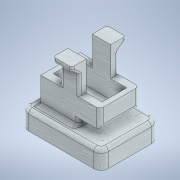
# Autodesk Inventor part: ramie 03-2
Saved by Autodesk Inventor 2021 (Build 250183000, 183)
## iProperties
Created: 2021-11-05
Part Number: ramie 03-2
Material: Generic
Document SubType Name: Modeling
Designer: Łukasz
Density: 1 g/cm^3
Appearance: Wood - Painted White
Author: Łukasz
Autodesk Inventor part; units mm, degrees
ref_plane "YZ Plane" through (0, 0, 0) normal (1, 0, 0) x (0, 1, 0)
ref_plane "XZ Plane" through (0, 0, 0) normal (0, 1, 0) x (-1, 0, 0)
ref_plane "XY Plane" through (0, 0, 0) normal (0, 0, 1) x (1, 0, 0)
sketch "Sketch1" plane through (0, 0, 0) normal (0, 0, 1) x (1, 0, 0)
  line L0 (0, 0) -> (-15, 0)
  line L1 (-15, 0) -> (-15, 39)
  line L2 (-15, 39) -> (0, 39)
  line L3 (0, 39) -> (0, 0)
  dimension "d0" = 15
  dimension "d1" = 39
  constraints: 8 end point, 2 parallel, 1 horizontal, 1 perpendicular
  measures "d0" distance of L1.end L2.end
  measures "d1" distance of L0.end L1.end
extrude "Extrusion1" add sketch "Sketch1" along normal blind 4
sketch "Sketch2" plane through (0, 0, 0) normal (1, 0, 0) x (0, 0, -1)
  line L0 (0, 39) -> (-4, 39) projected
  line L1 (0, 39) -> (8, 39)
  line L2 (0, 39) -> (0, 27)
  line L3 (0, 39) -> (0, 0) projected
  line L4 (8, 39) -> (8, 35)
  arc A0 (8, 35) -> (0, 27) centre (13.0554, 21.9446) ccw
  dimension "d5" = 8
  dimension "d6" = 12
  dimension "d7" = 4
  dimension "d8" = 14
  constraints: 6 end point, 2 point on circle, 1 centre point, 1 horizontal, 1 point on line, 1 vertical
  measures "d5" distance of L0.start L1.end
  measures "d6" distance of L0.start L2.end
  measures "d7" distance of L1.end L4.end
  measures "d8" radius of A0
extrude "Extrusion2" add sketch "Sketch2" against normal up to surface (15 mm away)
fillet "Fillet1" radius 3 1 edges at (-7.5, 35, -8)
ref_plane "Work Plane2" through (0, 0, 14) normal (0, 0, 1) x (1, 0, 0)
mirror "Mirror1" about plane through (0, 0, 14) normal (0, 0, 1) of "Extrusion1", "Extrusion2", "Fillet1"
sketch "Sketch3" plane through (-15, 0, 28) normal (0, -1, 0) x (1, 0, 0)
  line L0 (0, 0) -> (15, 0) projected
  line L1 (15, 0) -> (-12, 0)
  line L2 (-12, 0) -> (-12, -28)
  line L3 (-12, -28) -> (15, -28)
  line L4 (15, -28) -> (15, 0)
  point P0 (15, -28)
  dimension "d13" = 27
  dimension "d14" = 28
  constraints: 8 end point, 2 parallel, 1 horizontal, 1 perpendicular
  measures "d13" distance of L3.end L2.end
  measures "d14" distance of L2.end L1.end
extrude "Extrusion3" add sketch "Sketch3" along normal blind 4
sketch "Sketch4" plane through (-27, 0, 0) normal (-1, 0, 0) x (0, 0, 1)
  line L0 (0, 27) -> (0, -4) projected
  line L1 (0, -4) -> (28, -4)
  line L2 (28, -4) -> (28, 15)
  line L3 (28, 15) -> (0, 15)
  line L4 (0, 15) -> (0, -4)
  point P0 (0, 0)
  dimension "d17" = 28
  dimension "d18" = 19
  constraints: 8 end point, 2 parallel, 1 horizontal, 1 perpendicular
  measures "d17" distance of L3.end L2.end
  measures "d18" distance of L2.end L1.end
extrude "Extrusion4" add sketch "Sketch4" along normal blind 4
sketch "Sketch5" plane through (-15, 0, 28) normal (0, 1, 0) x (1, 0, 0)
  line L0 (0, 24) -> (15, 24) projected
  line L1 (-12, 28) -> (0, 28)
  line L2 (0, 28) -> (0, 24)
  line L3 (0, 24) -> (-12, 24)
  line L4 (-12, 24) -> (-12, 28)
  line L5 (15, 4) -> (0, 4) projected
  line L6 (0, 0) -> (-12, 0) projected
  line L7 (0, 4) -> (-12, 4)
  line L8 (-12, 4) -> (-12, 0)
  line L9 (-12, 0) -> (0, 0)
  line L10 (0, 0) -> (0, 4)
  point P0 (15, 28)
  constraints: 16 end point, 4 parallel, 2 horizontal, 2 perpendicular
extrude "Extrusion5" add sketch "Sketch5" along normal up to surface (15 mm away)
sketch "Sketch7" plane through (0, 39, 4) normal (1, 0, 0) x (0, 0, -1)
  line L0 (-20, -39) -> (0, -39) projected
  line L1 (-24, -24) -> (4, -24) projected
  line L2 (-20, -39) -> (-24, -39)
  line L3 (-24, -39) -> (-24, -24)
  line L4 (-24, -24) -> (-20, -24)
  line L5 (-20, -24) -> (-20, -39)
  line L6 (0, -39) -> (0, 0) projected
  line L7 (0, -24) -> (4, -24)
  line L8 (4, -24) -> (4, -39)
  line L9 (4, -39) -> (0, -39)
  line L10 (0, -39) -> (0, -24)
  point P0 (0, -24)
  constraints: 16 end point, 4 parallel, 2 horizontal, 2 perpendicular, 2 point on line
extrude "Extrusion6" add sketch "Sketch7" along normal blind 13 contours L2 L3 L1 L5 | L6 L1 L8 L9
sketch "Sketch8" plane through (13, 39, 4) normal (1, 0, 0) x (0, 0, -1)
  line L0 (4, -12) -> (4, -24) projected
  line L1 (-24, -43) -> (-24, -39) projected
  line L2 (4, -24) -> (-24, -24)
  line L3 (-24, -24) -> (-24, -43)
  line L4 (-24, -43) -> (4, -43)
  line L5 (4, -43) -> (4, -24)
  line L6 (4, -39) -> (0, -39) projected
  line L7 (4, -39) -> (-24, -39)
  constraints: 10 end point, 2 parallel, 1 collinear, 1 horizontal, 1 perpendicular
extrude "Extrusion7" add sketch "Sketch8" along normal blind 4 contours L3 L2 L5 L6 L7
sketch "Sketch10" plane through (-15, -4, 28) normal (0, -1, 0) x (1, 0, 0)
  line L0 (15, 0) -> (-16, 0) projected
  line L1 (-16, -28) -> (-16, 0) projected
  line L2 (15, -28) -> (-16, -28) projected
  line L3 (15, -28) -> (15, 0) projected
  point P0 (15, -28)
extrude "Extrusion8" add sketch "Sketch10" along normal blind 3
sketch "Sketch11" plane through (-15, 27, 28) normal (0, 0, 1) x (1, 0, 0)
  line L0 (0, 0) -> (15, 0) projected
  line L1 (0, 0) -> (0, -12) projected
  line L2 (0, -12) -> (-16, -12) projected
  line L3 (-16, -12) -> (-16, -34) projected
  line L4 (15, -34) -> (-16, -34) projected
  line L5 (15, -34) -> (15, -27) projected
  line L6 (15, -27) -> (32, -27) projected
  line L7 (32, -12) -> (32, -27) projected
  line L8 (15, -12) -> (32, -12) projected
  line L9 (15, -12) -> (15, 0) projected
  line L10 (15, -12) -> (15, 12) projected
  line L11 (0, 0) -> (15, 0)
  line L12 (15, 0) -> (15, 8.662)
  line L13 (15, 8.662) -> (0, 8.662)
  line L14 (0, 8.662) -> (0, 0)
  constraints: 8 end point, 2 parallel, 1 horizontal, 1 perpendicular, 1 point on line
extrude "Extrusion9" add sketch "Sketch11" along normal blind 2
sketch "Sketch12" plane through (0, 0, 0) normal (0, 0, -1) x (-1, 0, 0)
  line L0 (15, 27) -> (0, 27) projected
  line L1 (0, 27) -> (0, 15) projected
  line L2 (0, 15) -> (-17, 15) projected
  line L3 (-17, 0) -> (-17, 15) projected
  line L4 (0, 0) -> (-17, 0) projected
  line L5 (0, 0) -> (0, -7) projected
  line L6 (31, -7) -> (0, -7) projected
  line L7 (31, 15) -> (31, -7) projected
  line L8 (15, 15) -> (31, 15) projected
  line L9 (15, 27) -> (15, 15) projected
  line L10 (15, 27) -> (0, 27) projected
  line L11 (15, 39) -> (15, 15) projected
  line L12 (0, 27) -> (15, 27)
  line L13 (15, 27) -> (15, 35.9565)
  line L14 (15, 35.9565) -> (0, 35.9565)
  line L15 (0, 35.9565) -> (0, 27)
  constraints: 8 end point, 2 parallel, 1 horizontal, 1 perpendicular, 1 point on line
extrude "Extrusion10" add sketch "Sketch12" along normal blind 2
fillet "Fillet2" radius 2 16 edges at (0, 22.767, -2) (0, 35.3762, -7.5753) (0, 37.9575, -8) (0, 32.6347, -4.0153) (-15, 22.767, -2) (-15, 37.9575, -8) (-15, 32.6347, -4.0153) (-15, 35.3762, -7.5753) (0, 22.767, 30) (0, 35.3762, 35.5753) (0, 37.9575, 36) (0, 32.6347, 32.0153) (-15, 22.767, 30) (-15, 37.9575, 36) (-15, 32.6347, 32.0153) (-15, 35.3762, 35.5753)
sketch "Sketch14" plane through (-15, -7, 28) normal (0, -1, 0) x (1, 0, 0)
  circle A0 centre (-12.3388, -26.6572) radius 3.95
  circle A1 centre (-12.3388, -1.6572) radius 3.95
  circle A2 centre (30.6612, -1.6572) radius 3.95
  circle A3 centre (30.6612, -26.6572) radius 3.95
  line L0 (-3.3388, -18.1572) -> (-3.3388, -10.1572)
  line L1 (-3.3388, -10.1572) -> (21.6612, -10.1572)
  line L2 (21.6612, -10.1572) -> (21.6612, -18.1572)
  line L3 (21.6612, -18.1572) -> (-3.3388, -18.1572)
  arc A4 (44.5, 8.3428) -> (39.5, 13.5) centre (39.5025, 8.5) ccw
  line L4 (39.5, 13.5) -> (-23.5, 13.5)
  arc A5 (-23.5, 13.5) -> (-28.5, 8.5) centre (-23.5, 8.5) ccw
  line L5 (-28.5, 8.5) -> (-28.5, -36.5)
  arc A6 (-28.5, -36.5) -> (-23.5, -41.5) centre (-23.5, -36.5) ccw
  line L6 (-23.5, -41.5) -> (39.5, -41.5)
  arc A7 (39.5, -41.5) -> (44.5, -36.6572) centre (39.5025, -36.5) ccw
  line L7 (44.5, -36.6572) -> (44.5, 8.3428)
  line L8 (-16, -30) -> (-16, 2) projected
  line L9 (32, -30) -> (32, 2) projected
  line L10 (15, 2) -> (32, 2) projected
  line L11 (-18.5, 9.5) -> (34.5, 9.5)
  line L12 (40.5, 3.5) -> (40.5, -31.5)
  line L13 (34.5, -37.5) -> (-18.5, -37.5)
  line L14 (-24.5, -31.5) -> (-24.5, 3.5)
  arc A8 (40.5, 3.5) -> (34.5, 9.5) centre (34.5, 3.5) ccw
  arc A9 (-18.5, 9.5) -> (-24.5, 3.5) centre (-18.5, 3.5) ccw
  arc A10 (-24.5, -31.5) -> (-18.5, -37.5) centre (-18.5, -31.5) ccw
  arc A11 (34.5, -37.5) -> (40.5, -31.5) centre (34.5, -31.5) ccw
  point P0 (15, -28)
  point P1 (38.6612, -14.1572)
  dimension "d35" = 12.5
  dimension "d36" = 11.5
  dimension "d37" = 4
  dimension "d38" = 6
  dimension "d39" = 7.9
  dimension "d40" = 7.9
  dimension "d41" = 7.9
  dimension "d42" = 7.9
  constraints: 24 end point, 16 point on circle, 12 centre point, 8 tangent, 3 equal radius, 3 other
  measures "d35" distance between parallel lines of L7 L9
  measures "d36" distance between parallel lines of L10 L4
  measures "d37" distance between parallel lines of L4 L11
  measures "d38" radius of A8
  measures "d39" diameter of A2
  measures "d40" diameter of A3
  measures "d41" diameter of A1
  measures "d42" diameter of A0
extrude "Extrusion11" add sketch "Sketch14" along normal blind 15 contours L0 L1 L2 L3 | L11 A8 L12 A11 L13 A10 L14 A9
sketch "Sketch15" plane through (-15, -7, 28) normal (0, -1, 0) x (1, 0, 0)
  arc A0 (-10.2345, -30) -> (-16, -25.1746) centre (-12.3388, -26.6572) ccw projected
  circle A1 centre (-12.3388, -26.6572) radius 3.95
  arc A2 (-16, -3.1398) -> (-10.8463, 2) centre (-12.3388, -1.6572) ccw projected
  circle A3 centre (-12.3388, -1.6572) radius 3.95
  circle A4 centre (30.6612, -26.6572) radius 3.95 projected
  circle A5 centre (30.6612, -26.6572) radius 3.95
  circle A6 centre (30.6612, -1.6572) radius 3.95 projected
  circle A7 centre (30.6612, -1.6572) radius 3.95
  point P0 (15, -28)
  point P1 (-16, -25.1746)
  constraints: 4 centre point, 4 coincident
extrude "Extrusion12" add sketch "Sketch15" along normal blind 0.2
fillet "Fillet3" radius 3 11 edges at (-31, -7, 14) (-15.5, -7, -2) (-15.5, -7, 30) (-37.7426, -7, 35.7426) (-39.5, -7, 14) (-37.7426, -7, -7.7426) (-7, -7, -9.5) (23.7426, -7, -7.7426) (25.5, -7, 14) (23.7426, -7, 35.7426) (-7, -7, 37.5)
fillet "Fillet4" radius 3 7 edges at (17, 7.5, 30) (17, 7.5, -2) (17, 0, 14) (0, -6.1213, 30.8787) (0, -2, 30) (0, -6.1213, -2.8787) (0, -2, -2)
body "Solid1"
